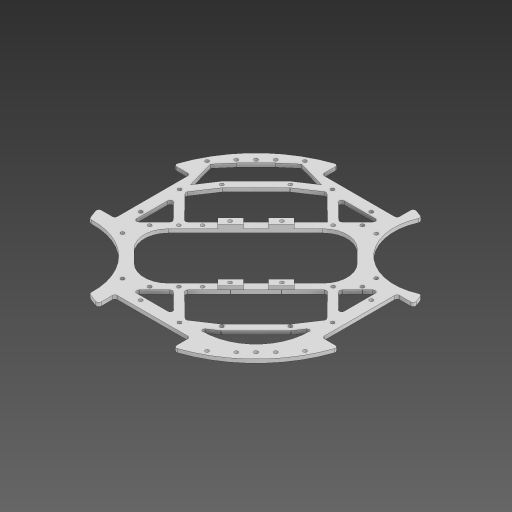
# Autodesk Inventor part: top_v2
Saved by Autodesk Inventor 2023 (Build 270158000, 158)
## iProperties
Created: 2025-06-24
Part Number: top_v2
Material: Типовые
Document SubType Name: Modeling
Designer: daa
Density: 1 g/cm^3
Appearance: По умолчанию
Author: daa
Autodesk Inventor part; units mm, degrees
(part 1 of 2)
ref_plane "YZ Plane" through (0, 0, 0) normal (1, 0, 0) x (0, 1, 0)
ref_plane "XZ Plane" through (0, 0, 0) normal (0, 1, 0) x (-1, 0, 0)
ref_plane "XY Plane" through (0, 0, 0) normal (0, 0, 1) x (1, 0, 0)
sketch "Эскиз1" plane through (0, 0, 0) normal (0, 1, 0) x (-1, 0, 0)
  line L0 (-79, -47.2724) -> (-79, 14.7276)
  line L1 (91.5447, -47.2724) -> (91.5447, 14.7276)
  line L2 (-79, -47.2724) -> (-93, -47.2724)
  line L3 (-79, 14.7276) -> (-93, 14.7276)
  line L4 (91.5447, -47.2724) -> (105.5447, -47.2724)
  line L5 (91.5447, 14.7276) -> (105.5447, 14.7276)
  line L6 (-24.7276, -101.5447) -> (37.2724, -101.5447)
  line L7 (-24.7276, 69) -> (37.2724, 69)
  line L8 (-24.7276, 69) -> (-24.7276, 83)
  line L9 (37.2724, 69) -> (37.2724, 83)
  line L10 (37.2724, -101.5447) -> (37.2724, -115.5447)
  line L11 (-24.7276, -101.5447) -> (-24.7276, -115.5447)
  arc A0 (-93, -47.2724) -> (-24.7276, -115.5447) centre (6.2724, -16.2724) ccw
  arc A1 (105.5447, 14.7276) -> (37.2724, 83) centre (6.2724, -16.2724) ccw
  arc A2 (-24.7276, 83) -> (-93, 14.7276) centre (6.2724, -16.2724) ccw
  arc A3 (37.2724, -115.5447) -> (105.5447, -47.2724) centre (6.2724, -16.2724) ccw
  dimension "d29" = 62
  dimension "d31" = 62
  dimension "d33" = 14
  dimension "d34" = 14
  dimension "d35" = 62
  dimension "d36" = 62
  dimension "d39" = 14
  dimension "d40" = 14
  constraints: 24 end point, 8 point on circle, 4 centre point, 4 horizontal, 3 parallel, 3 vertical, 2 point on line, 1 concentric
  measures "d29" distance of L0.start L0.end
  measures "d31" distance of L1.start L1.end
  measures "d33" distance of L0.end L3.end
  measures "d34" distance of L1.end L5.end
  measures "d35" distance of L6.start L6.end
  measures "d36" distance of L7.start L7.end
  measures "d39" distance of L7.start L8.end
  measures "d40" distance of L6.start L11.end
extrude "motor" add sketch "Эскиз1" along normal blind 3
sketch "Эскиз2" plane through (0, 3, 0) normal (0, 1, 0) x (1, 0, 0)
  arc A0 (24.7276, -83) -> (93, -14.7276) centre (-6.2724, 16.2724) ccw projected
  arc A1 (-37.2724, 115.5447) -> (-105.5447, 47.2724) centre (-6.2724, 16.2724) ccw projected
  circle A2 centre (-6.2724, 16.2724) radius 104
  line L0 (-6.2724, 16.2724) -> (-6.2724, -50.7276)
  arc A3 (-37.2724, 115.5447) -> (-105.5447, 47.2724) centre (-6.2724, 16.2724) ccw projected
  line L1 (-88.7917, -14.3063) -> (-40.8426, -62.2554)
  line L2 (-101.3809, -25.8032) -> (-48.3479, -78.8362)
  arc A4 (-105.5447, -14.7276) -> (-37.2724, -83) centre (-6.2724, 16.2724) ccw projected
  arc A5 (-48.3479, -78.8362) -> (-101.3809, -25.8032) centre (-98.035, -75.4903) ccw
  arc A6 (24.7276, -83) -> (93, -14.7276) centre (-6.2724, 16.2724) ccw projected
  line L3 (18.2427, 88.7365) -> (66.1918, 40.7874)
  line L4 (34.7276, 111.8495) -> (89.3048, 57.2724)
  arc A7 (34.7276, 111.8495) -> (89.3048, 57.2724) centre (70.9224, 93.4671) ccw
  line L5 (-91.5447, -14.7276) -> (-105.5447, -14.7276) projected
  arc A8 (-105.5447, -14.7276) -> (-101.3809, -25.8032) centre (-6.2724, 16.2724) ccw
  line L6 (-105.5447, -14.7276) -> (-80, -14.7276)
  line L7 (24.7276, 115.5447) -> (24.7276, 101.5447) projected
  line L8 (79, 47.2724) -> (93, 47.2724) projected
  arc A9 (89.3048, 57.2724) -> (34.7276, 111.8495) centre (-6.2724, 16.2724) ccw
  line L9 (93, 47.2724) -> (79, 47.2724)
  line L10 (24.7276, 115.5447) -> (24.7276, 101.5447)
  arc A10 (89.3048, 57.2724) -> (93, 47.2724) centre (-6.2724, 16.2724) ccw
  arc A11 (93, 47.2724) -> (24.7276, 115.5447) centre (-6.2724, 16.2724) ccw projected
  arc A12 (24.7276, 115.5447) -> (34.7276, 111.8495) centre (-6.2724, 16.2724) ccw
  line L11 (79, 47.2724) -> (59.7069, 47.2724)
  line L12 (24.7276, 101.5447) -> (24.7276, 82.2516)
  point P0 (0, 0)
  point P1 (-6.2724, -50.7276)
  point P2 (35.8032, 111.3809)
  point P3 (89.3048, 57.2724)
  point P4 (42.2173, 64.762)
  dimension "d181" = 208
  dimension "d190" = 67
  dimension "d205" = 75
  dimension "d207" = 17.0315
  dimension "d208" = 11.0756
  dimension "d209" = 104
  dimension "d316" = 28
  dimension "d317" = 10
  dimension "d318" = 10
  dimension "d330" = 40.5953
  constraints: 20 end point, 14 point on circle, 7 centre point, 4 point on line, 2 collinear, 2 tangent, 1 horizontal, 1 midpoint, 1 vertical
  measures "d181" diameter of A2
  measures "d190" distance of L0.end L0.start
  measures "d205" distance of L2.start L2.end
  measures "d207" distance between parallel lines of L1 L2
  measures "d208" horizontal distance of A2.end L2.end
  measures "d209" radius of A8
  measures "d316" distance from line of point (42.217, 64.762) L4
  measures "d317" distance from line of L7 L4.start
  measures "d318" distance from line of L4.end L8
  measures "d330" radius of A7
extrude "ball" cut sketch "Эскиз2" against normal blind 3 contours A2 L2 | L2 A5 | L4 A2 | A7 L4
sketch "Эскиз3" plane through (0, 3, 0) normal (0, 1, 0) x (1, 0, 0)
  arc A0 (93, 47.2724) -> (24.7276, 115.5447) centre (-6.2724, 16.2724) ccw projected
  line L0 (-6.2724, 16.2724) -> (97.7276, 16.2724) construction
  line L1 (67.2668, 89.8115) -> (-62.5447, -40)
  circle A1 centre (70.5306, -44.2673) radius 1.5
  circle A2 centre (54.2672, -60.5308) radius 1.5
  circle A3 centre (41.3053, -71.6104) radius 1.5
  circle A4 centre (81.6104, -31.3053) radius 1.5
  arc A5 (24.7276, -83) -> (93, -14.7276) centre (-6.2724, 16.2724) ccw projected
  line L2 (-6.2724, 16.2724) -> (97.7276, 16.2724) construction
  line L3 (-79.8115, 89.8115) -> (67.2668, -57.2668)
  line L4 (-91.5447, 47.2724) -> (-91.5447, -14.7276) projected
  line L5 (-91.5447, 16.2724) -> (79, 16.2724)
  line L6 (24.7276, 101.5447) -> (-37.2724, 101.5447) projected
  line L7 (-6.2724, 101.5447) -> (-6.2724, -69)
  line L8 (-6.2724, 101.5447) -> (-6.2724, -69)
  line L9 (-91.5447, 47.2724) -> (-91.5447, -14.7276) projected
  arc A6 (24.7276, -83) -> (93, -14.7276) centre (-6.2724, 16.2724) ccw projected
  circle A7 centre (-66.812, 93.0753) radius 1.5
  circle A8 centre (-83.0755, 76.8119) radius 1.5
  circle A9 centre (-94.1551, 63.85) radius 1.5
  circle A10 centre (-53.85, 104.1551) radius 1.5
  point P0 (0, 0)
  point P1 (67.2668, -57.2668)
  point P2 (67.2668, -57.2668)
  point P3 (-105.5447, 47.2724)
  point P4 (-79.8115, 89.8115)
  point P5 (-79.8115, 89.8115)
  point P6 (-79.8115, 89.8115)
  dimension "d65" = 3
  dimension "d66" = 3
  dimension "d67" = 3
  dimension "d68" = 3
  dimension "d69" = 23
  dimension "d71" = 57
  dimension "d74" = -12.962
  dimension "d78" = 25.9614
  constraints: 14 end point, 8 centre point, 8 symmetric about line, 4 point on circle, 3 midpoint, 2 horizontal, 2 vertical, 1 point on line, 4 other
  measures "d65" diameter of A1
  measures "d66" diameter of A2
  measures "d67" diameter of A3
  measures "d68" diameter of A4
  measures "d69" distance of A2.centre A1.centre
  measures "d71" distance of A3.centre A4.centre
  measures "d74" vertical distance of A1.centre A4.centre
  measures "d78" vertical distance of A4.centre point (67.267, -57.267)
extrude "hand_mount" cut sketch "Эскиз3" against normal blind 10
sketch "Эскиз5" plane through (0, 3, 0) normal (0, 1, 0) x (1, 0, 0)
  circle A0 centre (29.7645, -47.992) radius 1.5
  circle A1 centre (58.0485, -19.7074) radius 1.5
  circle A2 centre (-6.2982, 16.355) radius 104
  arc A3 (-105.5447, -14.7276) -> (-99.04, -30.7083) centre (-6.2982, 16.355) ccw projected
  line L0 (-6.2982, 16.355) -> (97.7018, 16.355) construction
  circle A4 centre (-71.4195, 53.192) radius 1.5
  circle A5 centre (-43.1349, 81.476) radius 1.5
  circle A6 centre (-45.0925, -54.9329) radius 1.5
  line L1 (-62.8214, -40.2767) -> (-61.356, -38.6694)
  line L2 (-61.356, -38.6694) -> (-45.4214, -38.6694) construction
  circle A7 centre (-77.6194, -22.406) radius 1.5
  arc A8 (24.7276, -83) -> (93, -14.7276) centre (-6.2724, 16.2724) ccw projected
  line L3 (-6.2982, 16.355) -> (97.7785, 16.355) construction
  line L4 (64.1086, -60.2947) -> (-82.2655, 87.2726)
  arc A9 (-37.2724, 115.5447) -> (-105.5447, 47.2724) centre (-6.2724, 16.2724) ccw projected
  circle A10 centre (27.3717, 81.7363) radius 1.5
  arc A11 (-48.3479, -78.8362) -> (-101.3809, -25.8032) centre (-98.035, -75.4903) ccw projected
  arc A12 (34.7276, 111.8495) -> (89.3048, 57.2724) centre (70.9224, 93.4671) ccw projected
  circle A13 centre (59.1841, 49.909) radius 1.5
  line L5 (27.3717, 81.7363) -> (71.0459, 81.7363) construction
  line L6 (27.3717, 81.7363) -> (59.1841, 49.909)
  line L7 (42.2173, 64.762) -> (43.2779, 65.8226)
  line L8 (42.2173, 64.762) -> (43.7173, 64.762) construction
  line L9 (-77.6194, -22.406) -> (-45.0925, -54.9329)
  line L10 (-77.6194, -22.406) -> (-31.6194, -22.406) construction
  point P0 (0, 0)
  point P1 (-62.8214, -40.2767)
  dimension "d116" = 3
  dimension "d117" = 3
  dimension "d118" = 40
  dimension "d119" = 208
  dimension "d121" = 64.347
  dimension "d126" = 3
  dimension "d130" = 2.175
  dimension "d332" = 45
  dimension "d335" = 1.5
  dimension "d336" = 45
  dimension "d337" = 46
  dimension "d338" = 45
  constraints: 22 end point, 9 centre point, 6 horizontal, 5 point on circle, 2 equal length, 2 midpoint, 1 coincident, 1 concentric, 1 symmetric about line, 1 other
  measures "d116" diameter of A0
  measures "d117" diameter of A1
  measures "d118" distance of A1.centre A0.centre
  measures "d119" diameter of A2
  measures "d121" vertical distance of L0.start A0.centre
  measures "d126" diameter of A6
  measures "d130" distance of L1.end L1.start
  measures "d332" distance of L5.start L6.end
  measures "d335" distance of L7.end L7.start
  measures "d336" angle of L8 L7
  measures "d337" distance of L9.start L9.end
  measures "d338" angle of L9 L10
extrude "Выдавливание5" cut sketch "Эскиз5" against normal blind 10 contours A0 | A1 | A4 | A5 | A6 | A7 | A10 | A13
sketch "Эскиз6" plane through (0, 3, 0) normal (0, 1, 0) x (1, 0, 0)
  circle A0 centre (-22.2724, 95.2947) radius 1.5
  circle A1 centre (9.7276, 95.2947) radius 1.5
  line L0 (24.7276, 115.5447) -> (24.7276, 101.5447) projected
  line L1 (24.7276, 101.5447) -> (-37.2724, 101.5447) projected
  circle A2 centre (-22.2724, -62.75) radius 1.5
  circle A3 centre (9.7276, -62.75) radius 1.5
  circle A4 centre (-85.2947, 32.2724) radius 1.5
  circle A5 centre (-85.2947, 0.2724) radius 1.5
  circle A6 centre (72.75, 32.2724) radius 1.5
  circle A7 centre (72.75, 0.2724) radius 1.5
  point P0 (0, 0)
  point P1 (24.7276, -69)
  point P2 (-37.2724, -69)
  point P3 (-91.5447, -14.7276)
  point P4 (-91.5447, 47.2724)
  point P5 (79, 47.2724)
  point P6 (79, -14.7276)
  dimension "d135" = 3
  dimension "d136" = 3
  dimension "d137" = 32
  dimension "d138" = 15
  dimension "d139" = 6.25
  dimension "d140" = 3
  dimension "d141" = 3
  dimension "d142" = 6.25
  dimension "d143" = 32
  dimension "d144" = 15
  dimension "d145" = 6.25
  dimension "d146" = 6.25
  dimension "d147" = 3
  dimension "d148" = 3
  dimension "d149" = 32
  dimension "d150" = 15
  dimension "d151" = 6.25
  dimension "d152" = 6.25
  dimension "d153" = 3
  dimension "d154" = 3
  dimension "d155" = 32
  dimension "d156" = 15
  dimension "d157" = 6.25
  dimension "d158" = 6.25
  constraints: 8 centre point
  measures "d135" diameter of A0
  measures "d136" diameter of A1
  measures "d137" distance of A1.centre A0.centre
  measures "d138" distance from line of L0 A1.centre
  measures "d139" distance from line of L1 A1.centre
  measures "d140" diameter of A2
  measures "d141" diameter of A3
  measures "d142" distance from line of L1 A0.centre
  measures "d143" distance of A2.centre A3.centre
  measures "d144" horizontal distance of point (24.728, -69) A3.centre
  measures "d145" vertical distance of point (24.728, -69) A3.centre
  measures "d146" vertical distance of point (-37.272, -69) A2.centre
  measures "d147" diameter of A4
  measures "d148" diameter of A5
  measures "d149" distance of A5.centre A4.centre
  measures "d150" vertical distance of A5.centre point (-91.545, -14.728)
  measures "d151" horizontal distance of A5.centre point (-91.545, -14.728)
  measures "d152" horizontal distance of A4.centre point (-91.545, 47.272)
  measures "d153" diameter of A6
  measures "d154" diameter of A7
  measures "d155" distance of A7.centre A6.centre
  measures "d156" vertical distance of point (79, 47.272) A6.centre
  measures "d157" horizontal distance of point (79, -14.728) A7.centre
  measures "d158" horizontal distance of point (79, 47.272) A6.centre
extrude "Выдавливание6" cut sketch "Эскиз6" against normal blind 10
fillet "Сопряжение1" radius 2 16 edges at (93, 1.5, -47.2724) (24.7276, 1.5, -115.5447) (24.7276, 1.5, -101.5447) (-37.2724, 1.5, -101.5447) (-37.2724, 1.5, -115.5447) (-105.5447, 1.5, -47.2724) (-91.5447, 1.5, -47.2724) (-91.5447, 1.5, 14.7276) (-105.5447, 1.5, 14.7276) (-37.2724, 1.5, 83) (-37.2724, 1.5, 69) (24.7276, 1.5, 69) (24.7276, 1.5, 83) (93, 1.5, 14.7276) (79, 1.5, 14.7276) (79, 1.5, -47.2724)
fillet "Сопряжение4" radius 2 4 edges at (-101.3809, 1.5, 25.8032) (-48.3479, 1.5, 78.8362) (34.7276, 1.5, -111.8495) (89.3048, 1.5, -57.2724)
sketch "Эскиз8" plane through (0, 3, 0) normal (0, 1, 0) x (1, 0, 0)
  circle A0 centre (62.3989, -52.3991) radius 1.6
  circle A1 centre (54.2672, -60.5308) radius 1.5
  circle A2 centre (54.2672, -60.5308) radius 1.5 projected
  line L0 (54.2672, -60.5308) -> (67.7672, -60.5308) construction
  circle A3 centre (70.5306, -44.2673) radius 1.5
  circle A4 centre (70.5306, -44.2673) radius 1.5 projected
  line L1 (70.5306, -44.2673) -> (82.0306, -44.2673) construction
  line L2 (70.5306, -44.2673) -> (60.52, -44.2673)
  circle A5 centre (70.5306, -44.2673) radius 1.5 projected
  line L3 (60.52, -44.2673) -> (70.5306, -44.2673)
  line L4 (70.5306, -44.2673) -> (62.3989, -52.3991)
  arc A6 (90.1213, 55.3142) -> (87.4532, 56.39) centre (88.2676, 54.5634) ccw projected
  arc A7 (33.8453, 109.9979) -> (87.4532, 56.39) centre (70.9224, 93.4671) ccw projected
  arc A8 (33.8453, 109.9979) -> (32.7695, 112.666) centre (32.0187, 110.8123) ccw projected
  arc A9 (32.7695, 112.666) -> (27.3747, 114.679) centre (-6.2724, 16.2724) ccw projected
  arc A10 (27.3747, 114.679) -> (24.7276, 112.7866) centre (26.7276, 112.7866) ccw projected
  line L5 (24.7276, 112.7866) -> (24.7276, 103.5447) projected
  arc A11 (22.7276, 101.5447) -> (24.7276, 103.5447) centre (22.7276, 103.5447) ccw projected
  line L6 (22.7276, 101.5447) -> (-35.2724, 101.5447) projected
  arc A12 (-37.2724, 103.5447) -> (-35.2724, 101.5447) centre (-35.2724, 103.5447) ccw projected
  line L7 (-37.2724, 103.5447) -> (-37.2724, 112.7866) projected
  arc A13 (-37.2724, 112.7866) -> (-39.9194, 114.679) centre (-39.2724, 112.7866) ccw projected
  arc A14 (-39.9194, 114.679) -> (-104.679, 49.9194) centre (-6.2724, 16.2724) ccw projected
  arc A15 (-104.679, 49.9194) -> (-102.7866, 47.2724) centre (-102.7866, 49.2724) ccw projected
  line L8 (-102.7866, 47.2724) -> (-93.5447, 47.2724) projected
  arc A16 (-91.5447, 45.2724) -> (-93.5447, 47.2724) centre (-93.5447, 45.2724) ccw projected
  line L9 (-91.5447, 45.2724) -> (-91.5447, -12.7276) projected
  arc A17 (-93.5447, -14.7276) -> (-91.5447, -12.7276) centre (-93.5447, -12.7276) ccw projected
  line L10 (-93.5447, -14.7276) -> (-102.7866, -14.7276) projected
  arc A18 (-102.7866, -14.7276) -> (-104.679, -17.3747) centre (-102.7866, -16.7276) ccw projected
  arc A19 (-104.679, -17.3747) -> (-101.9399, -24.5163) centre (-6.2724, 16.2724) ccw projected
  arc A20 (-101.9399, -24.5163) -> (-100.0204, -25.7303) centre (-100.1002, -23.7319) ccw projected
  arc A21 (-48.275, -77.4757) -> (-100.0204, -25.7303) centre (-98.035, -75.4903) ccw projected
  arc A22 (-48.275, -77.4757) -> (-47.061, -79.3952) centre (-46.2766, -77.5555) ccw projected
  arc A23 (-47.061, -79.3952) -> (-39.9194, -82.1343) centre (-6.2724, 16.2724) ccw projected
  arc A24 (-39.9194, -82.1343) -> (-37.2724, -80.2419) centre (-39.2724, -80.2419) ccw projected
  line L11 (-37.2724, -80.2419) -> (-37.2724, -71) projected
  arc A25 (-35.2724, -69) -> (-37.2724, -71) centre (-35.2724, -71) ccw projected
  line L12 (-35.2724, -69) -> (22.7276, -69) projected
  arc A26 (24.7276, -71) -> (22.7276, -69) centre (22.7276, -71) ccw projected
  line L13 (24.7276, -71) -> (24.7276, -80.2419) projected
  arc A27 (24.7276, -80.2419) -> (27.3747, -82.1343) centre (26.7276, -80.2419) ccw projected
  arc A28 (27.3747, -82.1343) -> (92.1343, -17.3747) centre (-6.2724, 16.2724) ccw projected
  arc A29 (92.1343, -17.3747) -> (90.2419, -14.7276) centre (90.2419, -16.7276) ccw projected
  line L14 (90.2419, -14.7276) -> (81, -14.7276) projected
  arc A30 (79, -12.7276) -> (81, -14.7276) centre (81, -12.7276) ccw projected
  line L15 (79, -12.7276) -> (79, 45.2724) projected
  arc A31 (81, 47.2724) -> (79, 45.2724) centre (81, 45.2724) ccw projected
  line L16 (81, 47.2724) -> (90.2419, 47.2724) projected
  arc A32 (90.2419, 47.2724) -> (92.1343, 49.9194) centre (90.2419, 49.2724) ccw projected
  arc A33 (92.1343, 49.9194) -> (90.1213, 55.3142) centre (-6.2724, 16.2724) ccw projected
  circle A34 centre (-94.1551, 63.85) radius 1.5 projected
  circle A35 centre (41.3053, -71.6104) radius 1.5 projected
  circle A36 centre (81.6104, -31.3053) radius 1.5 projected
  circle A37 centre (-53.85, 104.1551) radius 1.5 projected
  circle A38 centre (-83.0755, 76.8119) radius 1.5 projected
  circle A39 centre (54.2672, -60.5308) radius 1.5 projected
  circle A40 centre (70.5306, -44.2673) radius 1.5 projected
  circle A41 centre (-66.812, 93.0753) radius 1.5 projected
  circle A42 centre (-45.0925, -54.9329) radius 1.5 projected
  circle A43 centre (29.7645, -47.992) radius 1.5 projected
  circle A44 centre (-43.1349, 81.476) radius 1.5 projected
  circle A45 centre (27.3717, 81.7363) radius 1.5 projected
  circle A46 centre (-77.6194, -22.406) radius 1.5 projected
  circle A47 centre (58.0485, -19.7074) radius 1.5 projected
  circle A48 centre (-71.4195, 53.192) radius 1.5 projected
  circle A49 centre (-85.2947, 0.2724) radius 1.5 projected
  circle A50 centre (72.75, 0.2724) radius 1.5 projected
  circle A51 centre (-22.2724, 95.2947) radius 1.5 projected
  circle A52 centre (9.7276, -62.75) radius 1.5 projected
  circle A53 centre (-85.2947, 32.2724) radius 1.5 projected
  circle A54 centre (72.75, 32.2724) radius 1.5 projected
  circle A55 centre (9.7276, 95.2947) radius 1.5 projected
  circle A56 centre (-22.2724, -62.75) radius 1.5 projected
  line L17 (42.2173, 64.762) -> (-62.8214, -40.2767)
  arc A57 (-48.275, -77.4757) -> (-100.0204, -25.7303) centre (-98.035, -75.4903) ccw projected
  circle A58 centre (-74.9438, 84.9436) radius 1.6
  point P0 (0, 0)
  dimension "d212" = 3.2
  dimension "d216" = 3
  dimension "d221" = 3
  dimension "d311" = 11.5
  dimension "d312" = 45
  constraints: 12 end point, 4 centre point, 3 horizontal, 3 point on circle, 2 concentric, 1 coincident, 1 collinear, 1 symmetric about line, 1 other
  measures "d212" diameter of A0
  measures "d216" diameter of A1
  measures "d221" diameter of A3
  measures "d311" distance of L3.end L4.end
  measures "d312" angle of L3 L4
extrude "Выдавливание7" cut sketch "Эскиз8" against normal blind 10 contours A0 | A58
sketch "Эскиз9" plane through (0, 3, 0) normal (0, 1, 0) x (1, 0, 0)
  line L0 (-38.87, 27.5154) -> (-17.5154, 48.87)
  line L1 (-17.5154, 48.87) -> (26.3253, 5.0294)
  line L2 (26.3253, 5.0294) -> (4.9706, -16.3253)
  line L3 (4.9706, -16.3253) -> (-38.87, 27.5154)
  circle A0 centre (-6.2724, 16.2724) radius 104
  arc A1 (-39.9194, 114.679) -> (-104.679, 49.9194) centre (-6.2724, 16.2724) ccw projected
  circle A2 centre (-17.5154, 48.87) radius 1.5
  circle A3 centre (-38.87, 27.5154) radius 1.5
  circle A4 centre (4.9706, -16.3253) radius 1.5
  circle A5 centre (26.3253, 5.0294) radius 1.5
  point P0 (0, 0)
  dimension "d224" = 30.2
  dimension "d225" = 62
  dimension "d226" = 208
  dimension "d227" = 15.1
  dimension "d229" = 31
  dimension "d230" = 3
  dimension "d231" = 3
  dimension "d232" = 3
  dimension "d233" = 3
  constraints: 8 end point, 5 centre point, 4 coincident, 2 parallel, 1 concentric, 1 perpendicular
  measures "d224" distance of L1.end L2.end
  measures "d225" distance of L0.end L1.end
  measures "d226" diameter of A0
  measures "d227" distance from line of L1 A0.centre
  measures "d229" distance from line of L2 A0.centre
  measures "d230" diameter of A2
  measures "d231" diameter of A3
  measures "d232" diameter of A4
  measures "d233" diameter of A5
extrude "Выдавливание8" cut sketch "Эскиз9" against normal blind 10 contours L3 A3 L0 | L0 A3 L3 | A2 L1 L0 | L0 L1 A2 | A4 L2 L3 | L3 L2 A4 | A5 L2 L1 | L1 L2 A5
sketch "Эскиз10" plane through (0, 3, 0) normal (0, 1, 0) x (1, 0, 0)
  circle A0 centre (-6.2724, 16.2719) radius 104.0005
  arc A1 (-39.9194, 114.679) -> (-104.679, 49.9194) centre (-6.2724, 16.2724) ccw projected
  line L0 (-60.0125, 6.3729) -> (-72.0333, -5.648)
  line L1 (-72.0333, -5.648) -> (-28.1927, -49.4886)
  line L2 (-28.1927, -49.4886) -> (-16.1718, -37.4678)
  line L3 (-16.1718, -37.4678) -> (-60.0125, 6.3729)
  circle A2 centre (-60.0125, 6.3729) radius 1.5
  circle A3 centre (-72.0333, -5.648) radius 1.5
  circle A4 centre (-16.1718, -37.4678) radius 1.5
  circle A5 centre (-28.1927, -49.4886) radius 1.5
  arc A6 (27.3747, -82.1343) -> (92.1343, -17.3747) centre (-6.2724, 16.2724) ccw projected
  line L4 (-6.2724, 16.2724) -> (97.7276, 16.2724) construction
  line L5 (67.2668, -57.2668) -> (-79.8115, 89.8115)
  line L6 (3.6271, 70.0125) -> (15.648, 82.0333)
  line L7 (15.648, 82.0333) -> (59.4886, 38.1927)
  line L8 (59.4886, 38.1927) -> (47.4678, 26.1718)
  line L9 (47.4678, 26.1718) -> (3.6271, 70.0125)
  circle A7 centre (3.6271, 70.0125) radius 1.5
  circle A8 centre (15.648, 82.0333) radius 1.5
  circle A9 centre (47.4678, 26.1718) radius 1.5
  circle A10 centre (59.4886, 38.1927) radius 1.5
  point P0 (0, 0)
  point P1 (10, 10)
  point P2 (-6.2719, 16.2724)
  dimension "d248" = 17
  dimension "d249" = 62
  dimension "d250" = 9.899
  dimension "d251" = 45
  dimension "d252" = 3
  dimension "d253" = 3
  dimension "d254" = 3
  dimension "d255" = 3
  constraints: 20 end point, 10 symmetric about line, 9 centre point, 8 coincident, 2 parallel, 2 point on circle, 1 horizontal, 1 perpendicular, 1 tangent, 4 other
  measures "d248" distance of L2.end L1.end
  measures "d249" distance of L1.end L0.end
  measures "d250" vertical distance of L0.start A0.centre
  measures "d251" distance from line of L3 L4.start
  measures "d252" diameter of A2
  measures "d253" diameter of A3
  measures "d254" diameter of A4
  measures "d255" diameter of A5
extrude "Выдавливание9" cut sketch "Эскиз10" against normal blind 10 contours L3 A2 L0 | L0 A2 L3 | A3 L1 L0 | L0 L1 A3 | A4 L2 L3 | L3 L2 A4 | A5 L2 L1 | L1 L2 A5 | L9 A7 L6 | L6 A7 L9 | A8 L7 L6 | L6 L7 A8 | A9 L8 L9 | L9 L8 A9 | A10 L8 L7 | L7 L8 A10
sketch "Эскиз12" plane through (0, 3, 0) normal (0, 1, 0) x (1, 0, 0)
  circle A0 centre (-6.2724, 16.2724) radius 104
  arc A1 (27.3747, -82.1343) -> (92.1343, -17.3747) centre (-6.2724, 16.2724) ccw projected
  line L0 (-91.5447, 45.2724) -> (-91.5447, -12.7276) projected
  line L1 (-91.5447, 45.2724) -> (-91.5447, -12.7276) projected
  line L2 (79, -12.7276) -> (79, 45.2724) projected
  line L3 (22.7276, 101.5447) -> (-35.2724, 101.5447) projected
  line L4 (-35.2724, -69) -> (22.7276, -69) projected
  arc A2 (-48.275, -77.4757) -> (-100.0204, -25.7303) centre (-98.035, -75.4903) ccw projected
  arc A3 (33.8453, 109.9979) -> (87.4532, 56.39) centre (70.9224, 93.4671) ccw projected
  line L5 (-22.8893, -39.2355) -> (40.7503, 24.4041)
  line L6 (40.7503, 52.6884) -> (30.1437, 63.295)
  line L7 (1.8594, 63.295) -> (-61.7802, -0.3447)
  line L8 (-61.7802, -28.6289) -> (-51.1736, -39.2355)
  arc A4 (-51.1736, -39.2355) -> (-22.8893, -39.2355) centre (-37.0315, -25.0934) ccw
  arc A5 (-61.7802, -0.3447) -> (-61.7802, -28.6289) centre (-47.6381, -14.4868) ccw
  arc A6 (30.1437, 63.295) -> (1.8594, 63.295) centre (16.0015, 49.1528) ccw
  arc A7 (40.7503, 24.4041) -> (40.7503, 52.6884) centre (26.6081, 38.5462) ccw
  point P0 (-35.7144, -52.4142)
  point P1 (16.0015, 77.4371)
  point P2 (54.8924, 38.5462)
  point P3 (-75.9224, -14.4868)
  dimension "d302" = 208
  dimension "d323" = 130
  dimension "d324" = 55
  dimension "d325" = 69.65
  dimension "d328" = 20
  constraints: 9 tangent, 8 end point, 8 point on circle, 6 point on line, 5 centre point, 3 equal radius, 2 parallel, 1 perpendicular
  measures "d302" diameter of A0
  measures "d323" distance of point (-75.922, -14.487) point (16.002, 77.437)
  measures "d324" distance of point (16.002, 77.437) point (54.892, 38.546)
  measures "d325" horizontal distance of point (-75.922, -14.487) A0.centre
  measures "d328" radius of A4
extrude "Выдавливание10" cut sketch "Эскиз12" against normal blind 10 contours A4 L8 A5 L7 A6 L6 A7 L5
sketch "Эскиз14" plane through (0, 3, 0) normal (0, 1, 0) x (1, 0, 0)
  circle A0 centre (-28.1927, -49.4886) radius 1.5 projected
  circle A1 centre (-72.0333, -5.648) radius 1.5 projected
  circle A2 centre (-16.1718, -37.4678) radius 1.5 projected
  circle A3 centre (-60.0125, 6.3729) radius 1.5 projected
  circle A4 centre (4.9706, -16.3253) radius 1.5 projected
  circle A5 centre (-17.5154, 48.87) radius 1.5 projected
  circle A6 centre (26.3253, 5.0294) radius 1.5 projected
  circle A7 centre (-38.87, 27.5154) radius 1.5 projected
  circle A8 centre (62.3989, -52.3991) radius 1.6 projected
  arc A9 (90.1213, 55.3142) -> (87.4532, 56.39) centre (88.2676, 54.5634) ccw projected
  arc A10 (33.8453, 109.9979) -> (87.4532, 56.39) centre (70.9224, 93.4671) ccw projected
  arc A11 (33.8453, 109.9979) -> (32.7695, 112.666) centre (32.0187, 110.8123) ccw projected
  arc A12 (32.7695, 112.666) -> (27.3747, 114.679) centre (-6.2724, 16.2724) ccw projected
  arc A13 (27.3747, 114.679) -> (24.7276, 112.7866) centre (26.7276, 112.7866) ccw projected
  line L0 (24.7276, 112.7866) -> (24.7276, 103.5447) projected
  arc A14 (22.7276, 101.5447) -> (24.7276, 103.5447) centre (22.7276, 103.5447) ccw projected
  line L1 (22.7276, 101.5447) -> (-35.2724, 101.5447) projected
  arc A15 (-37.2724, 103.5447) -> (-35.2724, 101.5447) centre (-35.2724, 103.5447) ccw projected
  line L2 (-37.2724, 103.5447) -> (-37.2724, 112.7866) projected
  arc A16 (-37.2724, 112.7866) -> (-39.9194, 114.679) centre (-39.2724, 112.7866) ccw projected
  arc A17 (-39.9194, 114.679) -> (-104.679, 49.9194) centre (-6.2724, 16.2724) ccw projected
  arc A18 (-104.679, 49.9194) -> (-102.7866, 47.2724) centre (-102.7866, 49.2724) ccw projected
  line L3 (-102.7866, 47.2724) -> (-93.5447, 47.2724) projected
  arc A19 (-91.5447, 45.2724) -> (-93.5447, 47.2724) centre (-93.5447, 45.2724) ccw projected
  line L4 (-91.5447, 45.2724) -> (-91.5447, -12.7276) projected
  arc A20 (-93.5447, -14.7276) -> (-91.5447, -12.7276) centre (-93.5447, -12.7276) ccw projected
  line L5 (-93.5447, -14.7276) -> (-102.7866, -14.7276) projected
  arc A21 (-102.7866, -14.7276) -> (-104.679, -17.3747) centre (-102.7866, -16.7276) ccw projected
  arc A22 (-104.679, -17.3747) -> (-101.9399, -24.5163) centre (-6.2724, 16.2724) ccw projected
  arc A23 (-101.9399, -24.5163) -> (-100.0204, -25.7303) centre (-100.1002, -23.7319) ccw projected
  arc A24 (-48.275, -77.4757) -> (-100.0204, -25.7303) centre (-98.035, -75.4903) ccw projected
  arc A25 (-48.275, -77.4757) -> (-47.061, -79.3952) centre (-46.2766, -77.5555) ccw projected
  arc A26 (-47.061, -79.3952) -> (-39.9194, -82.1343) centre (-6.2724, 16.2724) ccw projected
  arc A27 (-39.9194, -82.1343) -> (-37.2724, -80.2419) centre (-39.2724, -80.2419) ccw projected
  line L6 (-37.2724, -80.2419) -> (-37.2724, -71) projected
  arc A28 (-35.2724, -69) -> (-37.2724, -71) centre (-35.2724, -71) ccw projected
  line L7 (-35.2724, -69) -> (22.7276, -69) projected
  arc A29 (24.7276, -71) -> (22.7276, -69) centre (22.7276, -71) ccw projected
  line L8 (24.7276, -71) -> (24.7276, -80.2419) projected
  arc A30 (24.7276, -80.2419) -> (27.3747, -82.1343) centre (26.7276, -80.2419) ccw projected
  arc A31 (27.3747, -82.1343) -> (92.1343, -17.3747) centre (-6.2724, 16.2724) ccw projected
  arc A32 (92.1343, -17.3747) -> (90.2419, -14.7276) centre (90.2419, -16.7276) ccw projected
  line L9 (90.2419, -14.7276) -> (81, -14.7276) projected
  arc A33 (79, -12.7276) -> (81, -14.7276) centre (81, -12.7276) ccw projected
  line L10 (79, -12.7276) -> (79, 45.2724) projected
  arc A34 (81, 47.2724) -> (79, 45.2724) centre (81, 45.2724) ccw projected
  line L11 (81, 47.2724) -> (90.2419, 47.2724) projected
  arc A35 (90.2419, 47.2724) -> (92.1343, 49.9194) centre (90.2419, 49.2724) ccw projected
  arc A36 (92.1343, 49.9194) -> (90.1213, 55.3142) centre (-6.2724, 16.2724) ccw projected
  circle A37 centre (-94.1551, 63.85) radius 1.5 projected
  circle A38 centre (41.3053, -71.6104) radius 1.5 projected
  circle A39 centre (81.6104, -31.3053) radius 1.5 projected
  circle A40 centre (-53.85, 104.1551) radius 1.5 projected
  circle A41 centre (-83.0755, 76.8119) radius 1.5 projected
  circle A42 centre (54.2672, -60.5308) radius 1.5 projected
  circle A43 centre (70.5306, -44.2673) radius 1.5 projected
  circle A44 centre (-66.812, 93.0753) radius 1.5 projected
  circle A45 centre (-45.0925, -54.9329) radius 1.5 projected
  circle A46 centre (29.7645, -47.992) radius 1.5 projected
  circle A47 centre (-43.1349, 81.476) radius 1.5 projected
  circle A48 centre (27.3717, 81.7363) radius 1.5 projected
  circle A49 centre (-77.6194, -22.406) radius 1.5 projected
  circle A50 centre (58.0485, -19.7074) radius 1.5 projected
  circle A51 centre (-71.4195, 53.192) radius 1.5 projected
  circle A52 centre (-85.2947, 0.2724) radius 1.5 projected
  circle A53 centre (72.75, 0.2724) radius 1.5 projected
  circle A54 centre (-22.2724, 95.2947) radius 1.5 projected
  circle A55 centre (9.7276, -62.75) radius 1.5 projected
  circle A56 centre (-85.2947, 32.2724) radius 1.5 projected
  circle A57 centre (72.75, 32.2724) radius 1.5 projected
  circle A58 centre (9.7276, 95.2947) radius 1.5 projected
  circle A59 centre (-22.2724, -62.75) radius 1.5 projected
  circle A60 centre (-43.1349, 81.476) radius 1.5 projected
  line L12 (-43.1349, 81.476) -> (-17.5154, 48.87)
  line L13 (-17.5154, 48.87) -> (-38.87, 27.5154)
  line L14 (-38.87, 27.5154) -> (-71.4195, 53.192)
  line L15 (-71.4195, 53.192) -> (-43.1349, 81.476)
  circle A61 centre (-71.4195, 53.192) radius 1.5 projected
  circle A62 centre (-38.87, 27.5154) radius 1.5 projected
  line L16 (-71.4195, 53.192) -> (-38.87, 27.5154) construction
  line L17 (-73.4324, 50.6403) -> (-40.8829, 24.9636)
  line L18 (-36.857, 30.0671) -> (-69.4065, 55.7437)
  arc A63 (-69.4065, 55.7437) -> (-73.4324, 50.6403) centre (-71.4195, 53.192) ccw
  arc A64 (-40.8829, 24.9636) -> (-36.857, 30.0671) centre (-38.87, 27.5154) ccw
  line L19 (-17.5154, 48.87) -> (-38.87, 27.5154) construction
  line L20 (-19.7968, 51.1514) -> (-41.1514, 29.7968)
  line L21 (-36.5885, 25.2339) -> (-15.2339, 46.5885)
  arc A65 (-15.2339, 46.5885) -> (-19.7968, 51.1514) centre (-17.5154, 48.87) ccw
  arc A66 (-41.1514, 29.7968) -> (-36.5885, 25.2339) centre (-38.87, 27.5154) ccw
  circle A67 centre (-17.5154, 48.87) radius 1.5 projected
  line L22 (-43.1349, 81.476) -> (-17.5154, 48.87) construction
  line L23 (-45.6905, 79.468) -> (-20.071, 46.862)
  line L24 (-14.9597, 50.878) -> (-40.5793, 83.484)
  arc A68 (-40.5793, 83.484) -> (-45.6905, 79.468) centre (-43.1349, 81.476) ccw
  arc A69 (-20.071, 46.862) -> (-14.9597, 50.878) centre (-17.5154, 48.87) ccw
  line L25 (-71.4195, 53.192) -> (-43.1349, 81.476) construction
  line L26 (-69.1213, 50.8938) -> (-40.8368, 79.1778)
  line L27 (-45.4331, 83.7742) -> (-73.7176, 55.4902)
  arc A70 (-73.7176, 55.4902) -> (-69.1213, 50.8938) centre (-71.4195, 53.192) ccw
  arc A71 (-40.8368, 79.1778) -> (-45.4331, 83.7742) centre (-43.1349, 81.476) ccw
  circle A72 centre (-22.2724, 95.2947) radius 1.5 projected
  arc A73 (-20.725, 48.5411) -> (-14.3057, 49.1989) centre (-17.5154, 48.87) ccw
  line L28 (-22.2724, 95.2947) -> (-43.1349, 81.476) construction
  line L29 (-24.0671, 98.0043) -> (-44.9297, 84.1856)
  line L30 (-41.3401, 78.7664) -> (-20.4776, 92.5851)
  arc A74 (-20.4776, 92.5851) -> (-24.0671, 98.0043) centre (-22.2724, 95.2947) ccw
  arc A75 (-44.9297, 84.1856) -> (-41.3401, 78.7664) centre (-43.1349, 81.476) ccw
  line L31 (-71.4195, 53.192) -> (-85.2947, 32.2724) construction
  line L32 (-74.128, 54.9885) -> (-88.0032, 34.0688)
  line L33 (-82.5862, 30.4759) -> (-68.711, 51.3956)
  arc A76 (-68.711, 51.3956) -> (-74.128, 54.9885) centre (-71.4195, 53.192) ccw
  arc A77 (-88.0032, 34.0688) -> (-82.5862, 30.4759) centre (-85.2947, 32.2724) ccw
  line L34 (-85.2947, 32.2724) -> (-60.0125, 6.3729) construction
  line L35 (-87.6204, 30.0021) -> (-62.3382, 4.1026)
  line L36 (-57.6867, 8.6432) -> (-82.969, 34.5426)
  arc A78 (-82.969, 34.5426) -> (-87.6204, 30.0021) centre (-85.2947, 32.2724) ccw
  arc A79 (-62.3382, 4.1026) -> (-57.6867, 8.6432) centre (-60.0125, 6.3729) ccw
  circle A80 centre (-60.0125, 6.3729) radius 1.5 projected
  line L37 (-60.0125, 6.3729) -> (-72.0333, -5.648) construction
  line L38 (-62.3106, 8.671) -> (-74.3315, -3.3498)
  line L39 (-69.7351, -7.9461) -> (-57.7143, 4.0747)
  arc A81 (-57.7143, 4.0747) -> (-62.3106, 8.671) centre (-60.0125, 6.3729) ccw
  arc A82 (-74.3315, -3.3498) -> (-69.7351, -7.9461) centre (-72.0333, -5.648) ccw
  line L40 (-72.0333, -5.648) -> (-85.2947, 0.2724) construction
  arc A83 (-73.3582, -8.6158) -> (-70.7084, -2.6802) centre (-72.0333, -5.648) ccw
  arc A84 (-83.9698, 3.2402) -> (-86.6196, -2.6954) centre (-85.2947, 0.2724) ccw
  line L41 (-85.2947, 0.2724) -> (-85.2947, 32.2724) construction
  line L42 (-82.0446, 0.2724) -> (-82.0446, 32.2724)
  line L43 (-88.5448, 32.2724) -> (-88.5448, 0.2724)
  arc A85 (-88.5448, 0.2724) -> (-82.0446, 0.2724) centre (-85.2947, 0.2724) ccw
  line L44 (-60.0125, 6.3729) -> (-38.87, 27.5154) construction
  line L45 (-41.1682, 29.8135) -> (-62.3106, 8.671)
  arc A86 (-62.3106, 8.671) -> (-57.7143, 4.0747) centre (-60.0125, 6.3729) ccw
  arc A87 (-36.5718, 25.2172) -> (-41.1682, 29.8135) centre (-38.87, 27.5154) ccw
  arc A88 (-82.2264, 1.3442) -> (-88.363, -0.7995) centre (-85.2947, 0.2724) ccw
  arc A89 (-68.9423, -6.6524) -> (-75.1243, -4.6435) centre (-72.0333, -5.648) ccw
  arc A90 (-20.2981, 50.5029) -> (-14.7326, 47.237) centre (-17.5154, 48.87) ccw
  circle A91 centre (-83.0755, 76.8119) radius 1.5 projected
  arc A92 (-80.1797, 78.2875) -> (-85.9713, 75.3363) centre (-83.0755, 76.8119) ccw
  arc A93 (-74.3153, 51.7164) -> (-68.5236, 54.6676) centre (-71.4195, 53.192) ccw
  arc A94 (-92.7338, 66.7729) -> (-95.5764, 60.9272) centre (-94.1551, 63.85) ccw
  arc A95 (-72.8408, 50.2691) -> (-69.9981, 56.1149) centre (-71.4195, 53.192) ccw
  line L46 (-83.0755, 76.8119) -> (-94.1551, 63.85) construction
  line L47 (-85.546, 78.9237) -> (-96.6257, 65.9618)
  line L48 (-91.6846, 61.7382) -> (-80.6049, 74.7001)
  arc A96 (-80.6049, 74.7001) -> (-85.546, 78.9237) centre (-83.0755, 76.8119) ccw
  arc A97 (-96.6257, 65.9618) -> (-91.6846, 61.7382) centre (-94.1551, 63.85) ccw
  arc A98 (-85.3757, 79.1121) -> (-80.7753, 74.5116) centre (-83.0755, 76.8119) ccw
  arc A99 (-64.5118, 90.7751) -> (-69.1123, 95.3755) centre (-66.812, 93.0753) ccw
  line L49 (-66.812, 93.0753) -> (-53.85, 104.1551) construction
  line L50 (-64.6984, 90.6026) -> (-51.7364, 101.6824)
  line L51 (-55.9637, 106.6279) -> (-68.9257, 95.5481)
  arc A100 (-68.9257, 95.5481) -> (-64.6984, 90.6026) centre (-66.812, 93.0753) ccw
  arc A101 (-51.7364, 101.6824) -> (-55.9637, 106.6279) centre (-53.85, 104.1551) ccw
  line L52 (-53.85, 104.1551) -> (-43.1349, 81.476) construction
  arc A102 (-50.9313, 105.5849) -> (-56.7687, 102.7253) centre (-53.85, 104.1551) ccw
  arc A103 (-46.0536, 80.0462) -> (-40.2162, 82.9058) centre (-43.1349, 81.476) ccw
  circle A104 centre (-94.1551, 63.85) radius 1.5 projected
  circle A105 centre (-85.2947, 32.2724) radius 1.5 projected
  line L53 (-97.2844, 62.972) -> (-88.424, 31.3943)
  line L54 (-82.1654, 33.1504) -> (-91.0259, 64.7281)
  arc A106 (-91.0259, 64.7281) -> (-97.2844, 62.972) centre (-94.1551, 63.85) ccw
  arc A107 (-88.424, 31.3943) -> (-82.1654, 33.1504) centre (-85.2947, 32.2724) ccw
  line L55 (-53.85, 104.1551) -> (-22.2724, 95.2947) construction
  line L56 (-54.7281, 101.0259) -> (-23.1504, 92.1654)
  line L57 (-21.3943, 98.424) -> (-52.972, 107.2844)
  arc A108 (-52.972, 107.2844) -> (-54.7281, 101.0259) centre (-53.85, 104.1551) ccw
  arc A109 (-23.1504, 92.1654) -> (-21.3943, 98.424) centre (-22.2724, 95.2947) ccw
  circle A110 centre (-85.2947, 0.2724) radius 1.5 projected
  circle A111 centre (-72.0333, -5.648) radius 1.5 projected
  line L58 (-85.2947, 0.2724) -> (-72.0333, -5.648) construction
  arc A112 (-83.9698, 3.2402) -> (-86.6196, -2.6954) centre (-85.2947, 0.2724) ccw
  arc A113 (-73.3582, -8.6158) -> (-70.7084, -2.6802) centre (-72.0333, -5.648) ccw
  line L59 (-72.0333, -5.648) -> (-85.2947, -18.9094) construction
  line L60 (-74.3315, -3.3498) -> (-87.5929, -16.6112)
  line L61 (-82.9965, -21.2076) -> (-69.7351, -7.9461)
  arc A114 (-69.7351, -7.9461) -> (-74.3315, -3.3498) centre (-72.0333, -5.648) ccw
  arc A115 (-87.5929, -16.6112) -> (-82.9965, -21.2076) centre (-85.2947, -18.9094) ccw
  line L62 (-85.2947, -18.9094) -> (-85.2947, 0.2724) construction
  line L63 (-82.0446, -18.9094) -> (-82.0446, 0.2724)
  line L64 (-88.5448, 0.2724) -> (-88.5448, -18.9094)
  arc A116 (-88.5448, -18.9094) -> (-82.0446, -18.9094) centre (-85.2947, -18.9094) ccw
  arc A117 (-82.0446, 0.2724) -> (-88.5448, 0.2724) centre (-85.2947, 0.2724) ccw
  arc A118 (-19.4919, 51.4201) -> (-15.5388, 46.3198) centre (-17.5154, 48.87) ccw
  circle A119 centre (-43.1349, 81.476) radius 1.5 projected
  arc A120 (-43.4289, 84.7128) -> (-42.8409, 78.2392) centre (-43.1349, 81.476) ccw
  circle A121 centre (-38.87, 27.5154) radius 1.5
  circle A122 centre (-17.5154, 48.87) radius 1.5
  line L65 (-15.2172, 46.5718) -> (26.2774, 88.0664)
  line L66 (21.681, 92.6627) -> (-19.8135, 51.1682)
  arc A123 (-19.8135, 51.1682) -> (-15.2172, 46.5718) centre (-17.5154, 48.87) ccw
  arc A124 (-39.9194, 114.679) -> (-104.679, 49.9194) centre (-6.2724, 16.2724) ccw
  line L67 (22.7276, 101.5447) -> (-35.2724, 101.5447) projected
  arc A125 (-22.2724, 98.5448) -> (-22.2724, 92.0446) centre (-22.2724, 95.2947) ccw
  line L68 (-37.2724, 92.0446) -> (-22.2724, 92.0446)
  line L69 (-37.2724, 103.5447) -> (-37.2724, 112.7866) projected
  arc A126 (-52.7875, 107.2266) -> (-54.9126, 101.0836) centre (-53.85, 104.1551) ccw
  arc A127 (-46.321, 82.37) -> (-39.9488, 80.582) centre (-43.1349, 81.476) ccw
  line L70 (-82.0446, 32.2724) -> (-82.0446, 47.2724)
  arc A128 (-37.2724, 92.0446) -> (-82.0446, 47.2724) centre (-38.3364, 48.3364) ccw
  circle A129 centre (-74.949, 84.9384) radius 1.6
  line L71 (-66.812, 93.0753) -> (-74.949, 84.9384) construction
  line L72 (-69.1123, 95.3755) -> (-77.2492, 87.2386)
  line L73 (-72.6487, 82.6382) -> (-64.5118, 90.7751)
  arc A130 (-64.5118, 90.7751) -> (-69.1123, 95.3755) centre (-66.812, 93.0753) ccw
  arc A131 (-77.2492, 87.2386) -> (-72.6487, 82.6382) centre (-74.949, 84.9384) ccw
  line L74 (-74.949, 84.9384) -> (-83.0755, 76.8119) construction
  line L75 (-77.2492, 87.2386) -> (-85.3757, 79.1121)
  line L76 (-80.7753, 74.5116) -> (-72.6487, 82.6382)
  arc A132 (-72.6487, 82.6382) -> (-77.2492, 87.2386) centre (-74.949, 84.9384) ccw
  arc A133 (-85.3757, 79.1121) -> (-80.7753, 74.5116) centre (-83.0755, 76.8119) ccw
  line L77 (-6.2724, 16.2724) -> (-79.8115, 89.8115)
  arc A134 (-39.9194, 114.679) -> (-104.679, 49.9194) centre (-6.2724, 16.2724) ccw projected
  line L78 (9.7276, 92.0446) -> (-22.2724, 92.0446)
  line L79 (-22.2724, 98.5448) -> (9.7276, 98.5448)
  line L80 (28.9094, 92.0446) -> (9.7276, 92.0446)
  line L81 (9.7276, 98.5448) -> (28.9094, 98.5448)
  arc A135 (28.9094, 92.0446) -> (28.9094, 98.5448) centre (28.9094, 95.2947) ccw
  circle A136 centre (15.648, 82.0333) radius 1.5 projected
  line L82 (15.648, 82.0333) -> (28.9094, 95.2947) construction
  line L83 (17.9481, 79.7332) -> (31.2095, 92.9946)
  line L84 (26.6093, 97.5948) -> (13.3479, 84.3334)
  arc A137 (13.3479, 84.3334) -> (17.9481, 79.7332) centre (15.648, 82.0333) ccw
  arc A138 (31.2095, 92.9946) -> (26.6093, 97.5948) centre (28.9094, 95.2947) ccw
  circle A139 centre (3.6271, 70.0125) radius 1.5 projected
  line L85 (-22.2724, 95.2947) -> (3.6271, 70.0125) construction
  line L86 (-24.5426, 92.969) -> (1.3568, 67.6867)
  line L87 (5.8974, 72.3382) -> (-20.0021, 97.6204)
  arc A140 (-20.0021, 97.6204) -> (-24.5426, 92.969) centre (-22.2724, 95.2947) ccw
  arc A141 (1.3568, 67.6867) -> (5.8974, 72.3382) centre (3.6271, 70.0125) ccw
  line L88 (-62.8214, -40.2767) -> (42.2173, 64.762)
  circle A142 centre (26.3253, 5.0294) radius 1.5
  line L89 (28.0956, -50.8877) -> (2.4189, -18.3382)
  line L90 (7.5224, -14.3123) -> (33.199, -46.8618)
  arc A143 (28.0956, -50.8877) -> (33.199, -46.8618) centre (30.6473, -48.8748) ccw
  arc A144 (7.5224, -14.3123) -> (2.4189, -18.3382) centre (4.9706, -16.3253) ccw
  line L91 (28.6067, 2.7479) -> (7.2521, -18.6067)
  line L92 (2.6892, -14.0438) -> (24.0438, 7.3108)
  arc A145 (28.6067, 2.7479) -> (24.0438, 7.3108) centre (26.3253, 5.0294) ccw
  arc A146 (2.6892, -14.0438) -> (7.2521, -18.6067) centre (4.9706, -16.3253) ccw
  line L93 (56.9233, -23.1458) -> (24.3173, 2.4738)
  line L94 (28.3333, 7.585) -> (60.9393, -18.0346)
  arc A147 (56.9233, -23.1458) -> (60.9393, -18.0346) centre (58.9313, -20.5902) ccw
  line L95 (28.3491, -46.5766) -> (56.6331, -18.292)
  line L96 (61.2295, -22.8884) -> (32.9455, -51.1729)
  arc A148 (28.3491, -46.5766) -> (32.9455, -51.1729) centre (30.6473, -48.8748) ccw
  arc A149 (26.6542, 8.239) -> (25.9964, 1.8197) centre (26.3253, 5.0294) ccw
  line L97 (75.4596, -1.5224) -> (61.6409, -22.385)
  line L98 (56.2217, -18.7954) -> (70.0404, 2.0671)
  arc A150 (75.4596, -1.5224) -> (70.0404, 2.0671) centre (72.75, 0.2724) ccw
  line L99 (32.4438, -51.5833) -> (11.5241, -65.4585)
  line L100 (7.9312, -60.0415) -> (28.8509, -46.1663)
  arc A151 (7.9312, -60.0415) -> (11.5241, -65.4585) centre (9.7276, -62.75) ccw
  line L101 (7.4574, -65.0757) -> (-18.4421, -39.7935)
  line L102 (-13.9016, -35.142) -> (11.9979, -60.4243)
  arc A152 (7.4574, -65.0757) -> (11.9979, -60.4243) centre (9.7276, -62.75) ccw
  line L103 (-13.8737, -39.7659) -> (-25.8945, -51.7868)
  line L104 (-30.4908, -47.1904) -> (-18.47, -35.1696)
  arc A153 (-13.8737, -39.7659) -> (-18.47, -35.1696) centre (-16.1718, -37.4678) ccw
  arc A154 (-30.4908, -47.1904) -> (-25.8945, -51.7868) centre (-28.1927, -49.4886) ccw
  arc A155 (-25.2402, -64.0749) -> (-19.3046, -61.4251) centre (-22.2724, -62.75) ccw
  line L105 (-22.2724, -59.4999) -> (9.7276, -59.4999)
  line L106 (9.7276, -66.0001) -> (-22.2724, -66.0001)
  arc A156 (-22.2724, -59.4999) -> (-22.2724, -66.0001) centre (-22.2724, -62.75) ccw
  line L107 (7.2688, -18.6234) -> (-13.8737, -39.7659)
  arc A157 (-18.47, -35.1696) -> (-13.8737, -39.7659) centre (-16.1718, -37.4678) ccw
  arc A158 (7.2688, -18.6234) -> (2.6725, -14.0271) centre (4.9706, -16.3253) ccw
  arc A159 (-23.3442, -65.8183) -> (-21.2005, -59.6817) centre (-22.2724, -62.75) ccw
  arc A160 (-27.1882, -52.5796) -> (-29.1972, -46.3976) centre (-28.1927, -49.4886) ccw
  circle A161 centre (54.2672, -60.5308) radius 1.5
  arc A162 (52.7916, -63.4266) -> (55.7428, -57.635) centre (54.2672, -60.5308) ccw
  arc A163 (32.1229, -45.9789) -> (29.1717, -51.7706) centre (30.6473, -48.8748) ccw
  line L108 (54.2672, -60.5308) -> (41.3053, -71.6104) construction
  line L109 (56.3789, -63.0013) -> (43.4171, -74.081)
  line L110 (39.1935, -69.1399) -> (52.1554, -58.0602)
  arc A164 (56.3789, -63.0013) -> (52.1554, -58.0602) centre (54.2672, -60.5308) ccw
  arc A165 (39.1935, -69.1399) -> (43.4171, -74.081) centre (41.3053, -71.6104) ccw
  line L111 (70.5306, -44.2673) -> (81.6104, -31.3053) construction
  line L112 (68.0579, -42.1536) -> (79.1377, -29.1916)
  line L113 (84.0832, -33.419) -> (73.0034, -46.381)
  arc A166 (68.0579, -42.1536) -> (73.0034, -46.381) centre (70.5306, -44.2673) ccw
  arc A167 (84.0832, -33.419) -> (79.1377, -29.1916) centre (81.6104, -31.3053) ccw
  arc A168 (80.1806, -34.224) -> (83.0402, -28.3866) centre (81.6104, -31.3053) ccw
  arc A169 (60.3611, -17.6715) -> (57.5015, -23.5089) centre (58.9313, -20.5902) ccw
  line L114 (40.4273, -74.7397) -> (8.8496, -65.8793)
  line L115 (10.6057, -59.6207) -> (42.1834, -68.4812)
  arc A170 (40.4273, -74.7397) -> (42.1834, -68.4812) centre (41.3053, -71.6104) ccw
  arc A171 (10.6057, -59.6207) -> (8.8496, -65.8793) centre (9.7276, -62.75) ccw
  line L116 (81.6104, -31.3053) -> (72.75, 0.2724) construction
  line L117 (78.4812, -32.1834) -> (69.6207, -0.6057)
  line L118 (75.8793, 1.1504) -> (84.7397, -30.4273)
  arc A172 (78.4812, -32.1834) -> (84.7397, -30.4273) centre (81.6104, -31.3053) ccw
  arc A173 (75.8793, 1.1504) -> (69.6207, -0.6057) centre (72.75, 0.2724) ccw
  line L119 (-28.1927, -49.4886) -> (-41.4541, -62.75) construction
  line L120 (-25.8945, -51.7868) -> (-39.1559, -65.0482)
  line L121 (-43.7523, -60.4518) -> (-30.4908, -47.1904)
  arc A174 (-25.8945, -51.7868) -> (-30.4908, -47.1904) centre (-28.1927, -49.4886) ccw
  arc A175 (-43.7523, -60.4518) -> (-39.1559, -65.0482) centre (-41.4541, -62.75) ccw
  line L122 (-41.4541, -62.75) -> (-22.2724, -62.75) construction
  line L123 (-41.4541, -59.4999) -> (-22.2724, -59.4999)
  line L124 (-22.2724, -66.0001) -> (-41.4541, -66.0001)
  arc A176 (-41.4541, -59.4999) -> (-41.4541, -66.0001) centre (-41.4541, -62.75) ccw
  arc A177 (-22.2724, -66.0001) -> (-22.2724, -59.4999) centre (-22.2724, -62.75) ccw
  arc A178 (55.6945, -20.2962) -> (62.1681, -20.8842) centre (58.9313, -20.5902) ccw
  circle A179 centre (4.9706, -16.3253) radius 1.5
  line L125 (24.0271, 7.3275) -> (65.5217, 48.8221)
  line L126 (70.118, 44.2257) -> (28.6234, 2.7312)
  arc A180 (24.0271, 7.3275) -> (28.6234, 2.7312) centre (26.3253, 5.0294) ccw
  arc A181 (69.4999, 0.2724) -> (76.0001, 0.2724) centre (72.75, 0.2724) ccw
  line L127 (69.4999, -14.7276) -> (69.4999, 0.2724)
  arc A182 (58.0373, -17.4041) -> (59.8253, -23.7763) centre (58.9313, -20.5902) ccw
  line L128 (9.7276, -59.4999) -> (24.7276, -59.4999)
  arc A183 (24.7276, -59.4999) -> (69.4999, -14.7276) centre (25.7917, -15.7917) ccw
  circle A184 centre (62.3937, -52.4043) radius 1.6
  line L129 (72.8308, -46.5676) -> (64.6939, -54.7045)
  line L130 (60.0934, -50.104) -> (68.2304, -41.9671)
  arc A185 (72.8308, -46.5676) -> (68.2304, -41.9671) centre (70.5306, -44.2673) ccw
  arc A186 (60.0934, -50.104) -> (64.6939, -54.7045) centre (62.3937, -52.4043) ccw
  line L131 (62.3937, -52.4043) -> (54.2672, -60.5308) construction
  line L132 (64.6939, -54.7045) -> (56.5674, -62.831)
  line L133 (51.9669, -58.2306) -> (60.0934, -50.104)
  arc A187 (64.6939, -54.7045) -> (60.0934, -50.104) centre (62.3937, -52.4043) ccw
  arc A188 (51.9669, -58.2306) -> (56.5674, -62.831) centre (54.2672, -60.5308) ccw
  line L134 (69.4999, 32.2724) -> (69.4999, 0.2724)
  line L135 (76.0001, 0.2724) -> (76.0001, 32.2724)
  line L136 (76.0001, 32.2724) -> (76.0001, 51.4541)
  arc A189 (76.0001, 51.4541) -> (69.4999, 51.4541) centre (72.75, 51.4541) ccw
  line L137 (69.4999, 51.4541) -> (69.4999, 32.2724)
  line L138 (57.1885, 40.4928) -> (70.4499, 53.7542)
  line L139 (75.0501, 49.154) -> (61.7887, 35.8926)
  arc A190 (57.1885, 40.4928) -> (61.7887, 35.8926) centre (59.4886, 38.1927) ccw
  arc A191 (75.0501, 49.154) -> (70.4499, 53.7542) centre (72.75, 51.4541) ccw
  line L140 (70.4243, -1.9979) -> (45.142, 23.9016)
  line L141 (49.7935, 28.4421) -> (75.0757, 2.5426)
  arc A192 (49.7935, 28.4421) -> (45.142, 23.9016) centre (47.4678, 26.1718) ccw
  point P0 (-55.1447, 40.3537)
  point P1 (-28.1927, 38.1927)
  point P2 (-30.3251, 65.173)
  point P3 (-32.7036, 88.3854)
  point P4 (-78.3571, 42.7322)
  point P5 (-72.6536, 19.3226)
  point P6 (-66.0229, 0.3625)
  point P7 (-78.664, -2.6878)
  point P8 (-85.2947, 16.2724)
  point P9 (-49.4412, 16.9441)
  point P10 (-81.3612, -10.9876)
  point P11 (-74.7305, -13.9478)
  point P12 (-88.6153, 70.3309)
  point P13 (-60.331, 98.6152)
  point P14 (-82.0446, 24.2901)
  point P15 (-64.5813, 6.4004)
  point P16 (-59.9846, 10.9971)
  point P17 (-43.7536, 27.2281)
  point P18 (-70.6616, 48.4546)
  point P19 (-81.135, 32.6639)
  point P20 (-38.4018, 80.7127)
  point P21 (-43.4272, 76.5874)
  point P22 (-66.5359, 53.4792)
  point P23 (-39.1066, 31.8416)
  point P24 (-21.8377, 49.1105)
  point P25 (-89.7249, 48.0612)
  point P26 (-57.7143, 4.0747)
  point P27 (-45.6905, 79.468)
  point P28 (-45.6905, 79.468)
  point P29 (-29.9864, 94.0836)
  point P30 (-84.082, 39.9808)
  point P31 (-78.664, -2.6878)
  point P32 (-78.664, -12.2787)
  point P33 (-85.2947, -9.3185)
  point P34 (-82.0446, -11.0629)
  point P35 (-5.6006, -26.8965)
  point P36 (-17.2231, 53.7586)
  point P37 (-85.6353, 78.8192)
  point P38 (-82.5862, 30.4759)
  point P39 (-20.4776, 92.5851)
  point P40 (-74.128, 54.9885)
  point P41 (-73.7176, 55.4902)
  point P42 (-45.4331, 83.7742)
  point P43 (-69.4065, 55.7437)
  point P44 (-73.4324, 50.6403)
  point P45 (-68.891, 51.1241)
  point P46 (-41.0678, 78.9468)
  point P47 (-40.5793, 83.484)
  point P48 (-40.5793, 83.484)
  point P49 (-73.4324, 50.6403)
  point P50 (-69.4065, 55.7437)
  point P51 (-20.071, 46.862)
  point P52 (-82.0446, 43.0526)
  point P53 (-33.0647, 92.0446)
  point P54 (-82.0446, 31.2925)
  point P55 (-70.8805, 89.0068)
  point P56 (-79.0122, 80.8751)
  point P57 (22.2787, 88.664)
  point P58 (-9.3226, 82.6536)
  point P59 (-14.2901, 92.0446)
  point P60 (3.5996, 74.5813)
  point P61 (13.2557, 84.2373)
  point P62 (21.0591, 92.0446)
  point P63 (-0.9971, 69.9846)
  point P64 (-22.6651, 91.1362)
  point P65 (78.5389, -32.3679)
  point P66 (69.4999, -10.52)
  point P67 (61.6409, -22.385)
  point P68 (61.2295, -22.8884)
  point P69 (32.4438, -51.5833)
  point P70 (20.5079, -59.4999)
  point P71 (69.4999, 43.6038)
  point P72 (61.6926, 35.8004)
  point P73 (52.0366, 26.1443)
  point P74 (69.4999, 8.2546)
  point P75 (58.168, -15.8571)
  point P76 (68.5915, -0.1204)
  point P77 (47.4399, 21.5476)
  point P78 (31.2139, 5.3216)
  point P79 (54.0427, -20.8825)
  point P80 (26.5658, 0.707)
  point P81 (9.2969, -16.5619)
  point P82 (30.9345, -43.9911)
  point P83 (10.1192, -58.5903)
  point P84 (25.9098, -48.1169)
  point P85 (4.6834, -21.2088)
  point P86 (-11.5476, -37.4399)
  point P87 (1.7454, -59.4999)
  point P88 (-16.1443, -42.0366)
  point P89 (-33.6076, -59.4999)
  point P90 (28.5794, -46.3463)
  point P91 (7.5288, -18.3301)
  point P92 (56.1929, -18.7322)
  point P93 (56.5654, -18.2765)
  point P94 (28.3301, 2.4712)
  point P95 (-40.8748, 30.0735)
  point P96 (-41.2769, 78.7376)
  point P97 (-20.0735, 50.8748)
  point P98 (-40.8212, 79.1101)
  point P99 (-80.7117, 74.5752)
  point P100 (-90.5571, 63.0573)
  point P101 (-53.0539, 100.5561)
  point P102 (-64.6017, 90.6852)
  dimension "d313" = 3.2
  constraints: 312 end point, 226 point on circle, 151 symmetric about line, 118 centre point, 80 tangent, 20 parallel, 19 midpoint, 11 concentric, 5 point on line, 2 collinear, 2 vertical, 1 perpendicular, 53 other